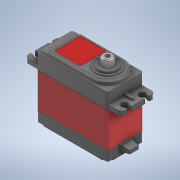
# Autodesk Inventor part: LF20MG
Saved by Autodesk Inventor 2020 (Build 240168000, 168)
## iProperties
Created: 2021-06-18
Part Number: LF20MG
Material: Plástico PC/ABS
Document SubType Name: Modeling
Designer: JCarlos
Density: 0.357273 g/cm^3
Appearance: Liso - Preto
Author: JCarlos
Autodesk Inventor part; units mm, degrees
ref_plane "YZ Plane" through (0, 0, 0) normal (1, 0, 0) x (0, 1, 0)
ref_plane "XZ Plane" through (0, 0, 0) normal (0, 1, 0) x (-1, 0, 0)
ref_plane "XY Plane" through (0, 0, 0) normal (0, 0, 1) x (1, 0, 0)
sketch "Esboço1" plane through (0, 0, 0) normal (0, 1, 0) x (-1, 0, 0)
  line L0 (20, 10) -> (-20, 10)
  line L1 (-20, 10) -> (-20, -10)
  line L2 (-20, -10) -> (20, -10)
  line L3 (20, -10) -> (20, 10)
  line L4 (20, 10) -> (-20, -10) construction
  line L5 (-20, 10) -> (20, -10) construction
  point P0 (0, 0)
  dimension "d0" = 40
  dimension "d1" = 20
  constraints: 12 end point, 2 midpoint, 2 parallel, 1 horizontal, 1 perpendicular
  measures "d0" distance of L1.end L2.end
  measures "d1" distance of L0.end L1.end
extrude "Extrusão1" add sketch "Esboço1" along normal blind 38
sketch "Esboço2" plane through (20, 0, 10) normal (1, 0, 0) x (0, 0, -1)
  line L0 (0.5, 29.25) -> (19.5, 29.25)
  line L1 (19.5, 29.25) -> (19.5, 26.75)
  line L2 (19.5, 26.75) -> (0.5, 26.75)
  line L3 (0.5, 26.75) -> (0.5, 29.25)
  line L4 (0.5, 29.25) -> (19.5, 26.75) construction
  line L5 (19.5, 29.25) -> (0.5, 26.75) construction
  line L6 (20, 0) -> (20, 38) projected
  line L7 (0, 0) -> (0, 38) projected
  line L8 (0, 0) -> (20, 0) projected
  point P0 (10, 0)
  point P1 (10, 28)
  dimension "d4" = 26.75
  dimension "d5" = 2.5
  dimension "d25" = 19
  dimension "d26" = 10
  constraints: 12 end point, 2 midpoint, 2 parallel, 1 horizontal, 1 perpendicular
  measures "d4" distance between parallel lines of L8 L2
  measures "d5" distance between parallel lines of L2 L0
  measures "d25" distance of L0.start L0.end
  measures "d26" distance from line of L7 point (10, 28)
extrude "Extrusão2" add sketch "Esboço2" along normal blind 7.25
sketch "Esboço3" plane through (20, 29.25, 9.5) normal (0, 1, 0) x (1, 0, 0)
  circle A0 centre (4.5, 4.5) radius 1.875
  circle A1 centre (4.5, 14.5) radius 1.875
  line L0 (0, 19) -> (0, 0) projected
  line L1 (0, 9.5) -> (2.4231, 9.5)
  line L2 (-20, 23.5) -> (-20, -4.5) projected
  line L3 (5.8975, 15.75) -> (7.25, 15.75)
  line L4 (7.25, 0) -> (7.25, 19) projected
  line L5 (5.8975, 13.25) -> (7.25, 13.25)
  line L6 (7.25, 15.75) -> (7.25, 13.25)
  line L7 (5.8975, 5.75) -> (7.25, 5.75)
  line L8 (5.8975, 3.25) -> (7.25, 3.25)
  line L9 (7.25, 3.25) -> (7.25, 5.75)
  point P0 (-20, 9.5)
  dimension "d8" = 3.75
  dimension "d9" = 10
  dimension "d10" = 5
  dimension "d11" = 24.5
  dimension "d12" = 2.5
  dimension "d13" = 1.25
  dimension "d14" = 2.5
  dimension "d15" = 1.25
  constraints: 14 end point, 4 point on circle, 3 horizontal, 3 perpendicular, 3 point on line, 2 centre point, 1 collinear, 1 equal radius, 1 midpoint, 1 vertical alignment
  measures "d8" diameter of A1
  measures "d9" distance of A1.centre A0.centre
  measures "d10" vertical distance of L1.end A0.centre
  measures "d11" distance from line of L2 A0.centre
  measures "d12" distance between parallel lines of L5 L3
  measures "d13" distance from line of A1.centre L3
  measures "d14" distance between parallel lines of L8 L7
  measures "d15" distance from line of A0.centre L7
extrude "Extrusão3" cut sketch "Esboço3" against normal through all
sketch "Esboço5" plane through (20, 29.25, 9.5) normal (0, 1, 0) x (1, 0, 0)
  line L0 (0, 10.5) -> (4, 10.5)
  line L1 (5, 9.5) -> (5, 9.5)
  line L2 (4, 8.5) -> (0, 8.5)
  line L3 (0, 8.5) -> (0, 10.5)
  line L4 (0, -0.5) -> (0, 19.5) projected
  arc A0 (5, 9.5) -> (4, 10.5) centre (4, 9.5) ccw
  arc A1 (4, 8.5) -> (5, 9.5) centre (4, 9.5) ccw
  line L5 (16.7, 9.5) -> (-49.45, 9.5) projected
  point P0 (-20, 9.5)
  point P1 (5, 8.5)
  point P2 (5, 10.5)
  point P3 (5, 9.5)
  dimension "d19" = 5
  dimension "d20" = 2
  dimension "d21" = 1
  dimension "d22" = 1
  constraints: 8 end point, 4 point on circle, 4 point on line, 4 tangent, 2 centre point, 2 parallel, 1 collinear, 1 concentric, 1 horizontal, 1 perpendicular
  measures "d19" distance of L0.start point (5, 10.5)
  measures "d20" distance of point (5, 10.5) point (5, 8.5)
  measures "d21" radius of A0
  measures "d22" distance between parallel lines of L5 L0
extrude "Extrusão4" add sketch "Esboço5" along normal blind 1
sketch "Esboço6" plane through (0, 38, 0) normal (0, 1, 0) x (1, 0, 0)
  line L0 (-19.25, 9.25) -> (10, 9.25)
  line L1 (19.25, 0) -> (19.25, 0)
  line L2 (10, -9.25) -> (-19.25, -9.25)
  line L3 (-19.25, -9.25) -> (-19.25, 9.25)
  arc A0 (19.25, 0) -> (10, 9.25) centre (10, 0) ccw
  arc A1 (10, -9.25) -> (19.25, 0) centre (10, 0) ccw
  line L4 (20, 10) -> (-20, 10) projected
  line L5 (20, -10) -> (20, 10) projected
  line L6 (-20, 10) -> (20, 10)
  line L7 (20, 10) -> (20, -10)
  line L8 (20, -10) -> (-20, -10)
  line L9 (-20, -10) -> (-20, 10)
  point P0 (0, 0)
  point P1 (19.25, 9.25)
  point P2 (-19.25, 0)
  point P3 (19.25, 0)
  dimension "d28" = 38.5
  dimension "d29" = 18.5
  dimension "d30" = 9.25
  dimension "d31" = 19.25
  constraints: 16 end point, 4 parallel, 4 point on circle, 4 tangent, 2 centre point, 2 horizontal, 2 perpendicular, 2 point on line, 1 concentric, 1 horizontal alignment, 1 midpoint
  measures "d28" distance of L0.start point (19.25, 9.25)
  measures "d29" distance of L2.end L0.start
  measures "d30" radius of A0
  measures "d31" distance of point (0, 0) L1.start
extrude "Extrusão5" cut sketch "Esboço6" against normal blind 2.5
sketch "Esboço7" plane through (0, 38, 0) normal (0, 1, 0) x (1, 0, 0)
  line L0 (-19.25, 9.25) -> (-19.25, -9.25) projected
  line L1 (-19.25, 9.25) -> (-15.25, 9.25)
  line L2 (-15.25, 9.25) -> (-15.25, -9.25)
  line L3 (-15.25, -9.25) -> (-19.25, -9.25)
  line L4 (-19.25, -9.25) -> (-19.25, 9.25)
  line L5 (-19.25, -9.25) -> (10, -9.25) projected
  point P0 (0, 0)
  dimension "d34" = 4
  constraints: 8 end point, 2 parallel, 1 collinear, 1 horizontal, 1 perpendicular
  measures "d34" distance of L0.start L1.end
extrude "Extrusão6" cut sketch "Esboço7" against normal blind 1.5
sketch "Esboço8" plane through (0, 38, 0) normal (0, 1, 0) x (1, 0, 0)
  circle A0 centre (10, 0) radius 6.75
  arc A1 (10, -9.25) -> (10, 9.25) centre (10, 0) ccw projected
  point P0 (0, 0)
  dimension "d37" = 13.5
  dimension "d38" = 10
  constraints: 1 centre point, 1 concentric, 1 horizontal alignment
  measures "d37" diameter of A0
  measures "d38" distance of point (0, 0) A0.centre
extrude "Extrusão7" add sketch "Esboço8" along normal blind 0.5
sketch "Esboço9" plane through (10, 38.5, 0) normal (0, 1, 0) x (1, 0, 0)
  circle A0 centre (0, 0) radius 5.5
  circle A1 centre (0, 0) radius 6.75 projected
  point P0 (-10, 0)
  dimension "d41" = 11
  constraints: 1 centre point, 1 concentric
  measures "d41" diameter of A0
extrude "Extrusão8" add sketch "Esboço9" along normal blind 1 contours A0
sketch "Esboço10" plane through (10, 39.5, 0) normal (0, 1, 0) x (1, 0, 0)
  circle A0 centre (0, 0) radius 2.95
  circle A1 centre (0, 0) radius 5.5 projected
  point P0 (-10, 0)
  dimension "d44" = 5.9
  constraints: 1 centre point, 1 concentric
  measures "d44" diameter of A0
extrude "Extrusão9" add sketch "Esboço10" along normal blind 4 contours A0
sketch "Esboço11" plane through (0, 0, 0) normal (0, -1, 0) x (1, 0, 0)
  line L0 (20, 10) -> (-20, 10) projected
  line L1 (20, 10) -> (16, 10)
  line L2 (16, 10) -> (16, 8.5)
  line L3 (18.5, 6) -> (20, 6)
  line L4 (20, 6) -> (20, 10)
  arc A0 (16, 8.5) -> (18.5, 6) centre (18.5, 8.5) ccw
  point P0 (0, 0)
  dimension "d47" = 4
  dimension "d48" = 4
  dimension "d49" = 2.5
  constraints: 8 end point, 2 parallel, 2 point on circle, 2 tangent, 1 centre point, 1 horizontal, 1 perpendicular
  measures "d47" distance of L3.end L0.start
  measures "d48" distance between parallel lines of L2 L4
  measures "d49" radius of A0
extrude "Extrusão10" cut sketch "Esboço11" against normal blind 1.5
mirror "Espelhamento1" about plane through (0, 0, 0) normal (0, 0, 1) of "Extrusão10"
mirror "Espelhamento2" about plane through (0, 0, 0) normal (1, 0, 0) of "Extrusão10", "Espelhamento1"
mirror "Espelhamento3" about plane through (0, 0, 0) normal (1, 0, 0) of "Extrusão2", "Extrusão3", "Extrusão4"
sketch "Esboço12" plane through (20, 35.5, 10) normal (1, 0, 0) x (0, 0, -1)
  line L0 (6.5, -28.5) -> (13.5, -28.5)
  line L1 (13.5, -28.5) -> (13.5, -32.5)
  line L2 (13.5, -32.5) -> (6.5, -32.5)
  line L3 (6.5, -32.5) -> (6.5, -28.5)
  line L4 (4, -35.5) -> (16, -35.5) projected
  point P0 (10, -35.5)
  point P1 (10, -32.5)
  point P2 (10, -35.5)
  dimension "d52" = 7
  dimension "d53" = 4
  dimension "d54" = 3
  constraints: 8 end point, 2 midpoint, 2 parallel, 1 horizontal, 1 perpendicular, 1 vertical alignment
  measures "d52" distance of L0.start L0.end
  measures "d53" distance of L2.end L0.start
  measures "d54" distance between parallel lines of L4 L2
extrude "Extrusão11" add sketch "Esboço12" along normal blind 1
sketch "Esboço13" plane through (21, 35.5, 10) normal (1, 0, 0) x (0, 0, -1)
  line L0 (13.5, -32.5) -> (13.5, -28.5) projected
  line L1 (13.5, -28.5) -> (6.5, -28.5) projected
  line L2 (6.5, -28.5) -> (6.5, -32.5) projected
  line L3 (6.5, -32.5) -> (13.5, -32.5) projected
  line L4 (7, -29) -> (13, -29)
  line L5 (13, -29) -> (13, -32)
  line L6 (13, -32) -> (7, -32)
  line L7 (7, -32) -> (7, -29)
  point P0 (10, -35.5)
  dimension "d57" = 6
  constraints: 8 end point, 3 other
  measures "d57" distance of L4.start L4.end
extrude "Extrusão12" add sketch "Esboço13" along normal blind 4 draft -8 contours L4 L5 L6 L7
fillet "Arredondamento2" radius 1 6 edges at (20, 18.5, 10) (-20, 18.5, 10) (20, 18.5, -10) (-20, 18.5, -10) (-19.25, 36, 9.25) (-19.25, 36, -9.25)
sketch "Esboço15" plane through (0, 0, 0) normal (0, 0, 1) x (1, 0, 0)
  line L0 (20.1, 26.75) -> (20, 26.75)
  line L1 (20, 26.75) -> (20, 7)
  line L2 (20, 7) -> (20.1, 7)
  line L3 (20.1, 7) -> (20.1, 26.75)
  line L4 (20, 26.75) -> (20, 1.5) projected
  line L5 (19.866, 26.75) -> (27.25, 26.75) projected
  line L6 (20, 7) -> (21, 7) projected
  point P0 (0, 0)
  dimension "d61" = 0.1
  constraints: 8 end point, 3 collinear, 2 parallel, 1 horizontal, 1 perpendicular
  measures "d61" distance between parallel lines of L1 L3
sketch3d "Esboço 3D1"
  line L0 (20, 35.5, 9) -> (20, 35.5, -9)
  arc A0 (20, 35.5, -9) -> (19, 35.5, -10) centre (19, 35.5, -9) ccw
  line L1 (19, 35.5, -10) -> (-19, 35.5, -10)
  arc A1 (-19, 35.5, -10) -> (-20, 35.5, -9) centre (-19, 35.5, -9) ccw
  line L2 (-20, 35.5, -9) -> (-20, 35.5, 9)
  arc A2 (-20, 35.5, 9) -> (-19, 35.5, 10) centre (-19, 35.5, 9) ccw
  line L3 (-19, 35.5, 10) -> (19, 35.5, 10)
  arc A3 (19, 35.5, 10) -> (20, 35.5, 9) centre (19, 35.5, 9) ccw
sweep "Varredura1" add profiles "Esboço15" path "Esboço 3D1"
chamfer "Chanfro1" distance 1 angle 45 7 edges at (0, 0, 10) (-20, 0, 0) (0, 0, -10) (20, 0, 0) (-2.625, 38, 9.25) (19.25, 38, 0) (-2.625, 38, -9.25)
chamfer "Chanfro2" distance 1.5 angle 45 1 edges at (-15.25, 38, 0)
fillet "Arredondamento3" radius 2 4 edges at (-27.25, 28, 9.5) (-27.25, 28, -9.5) (27.25, 28, 9.5) (27.25, 28, -9.5)
sketch "Esboço16" plane through (0, 38, 0) normal (0, 1, 0) x (1, 0, 0)
  line L0 (1, 7.5) -> (-12, 7.5)
  line L1 (-13, 6.5) -> (-13, -6.5)
  line L2 (-12, -7.5) -> (1, -7.5)
  line L3 (2, -6.5) -> (2, 6.5)
  line L4 (-13.75, -8.25) -> (-13.75, 8.25) projected
  arc A0 (2, 6.5) -> (1, 7.5) centre (1, 6.5) ccw
  arc A1 (1, -7.5) -> (2, -6.5) centre (1, -6.5) ccw
  arc A2 (-13, -6.5) -> (-12, -7.5) centre (-12, -6.5) ccw
  arc A3 (-12, 7.5) -> (-13, 6.5) centre (-12, 6.5) ccw
  point P0 (0, 0)
  point P1 (2, 7.5)
  point P2 (-13, -7.5)
  point P3 (2, -7.5)
  point P4 (2, 0)
  dimension "d71" = 15
  dimension "d72" = 15
  dimension "d73" = 0.75
  dimension "d74" = 1
  constraints: 8 end point, 8 point on circle, 8 tangent, 6 point on line, 4 centre point, 3 equal radius, 2 parallel, 1 horizontal, 1 horizontal alignment, 1 midpoint, 1 perpendicular
  measures "d71" distance of point (2, -7.5) point (2, 7.5)
  measures "d72" distance of point (-13, -7.5) point (2, -7.5)
  measures "d73" distance between parallel lines of L1 L4
  measures "d74" radius of A0
extrude "Extrusão13" cut sketch "Esboço16" against normal blind 0.2
sketch "Esboço17" plane through (10, 43.5, 0) normal (0, 1, 0) x (1, 0, 0)
  circle A0 centre (0, 0) radius 1.25
  circle A1 centre (0, 0) radius 2.95 projected
  point P0 (-10, 0)
  dimension "d77" = 2.5
  constraints: 1 centre point, 1 concentric
  measures "d77" diameter of A0
extrude "Extrusão14" cut sketch "Esboço17" against normal blind 5 contours A0
chamfer "Chanfro3" distance 0.5 angle 45 1 edges at (7.05, 43.5, 0)
equation "\"d26\" = 0.5 * d1"
equation "\"d10\" = 0.5 * d9"
equation "\"d13\" = 0.5 * d12"
equation "\"d14\" = d12"
equation "\"d15\" = 0.5 * d14"
equation "\"d22\" = 0.5 * d20"
equation "\"d31\" = 0.5 * d28"
equation "\"d48\" = d47"
